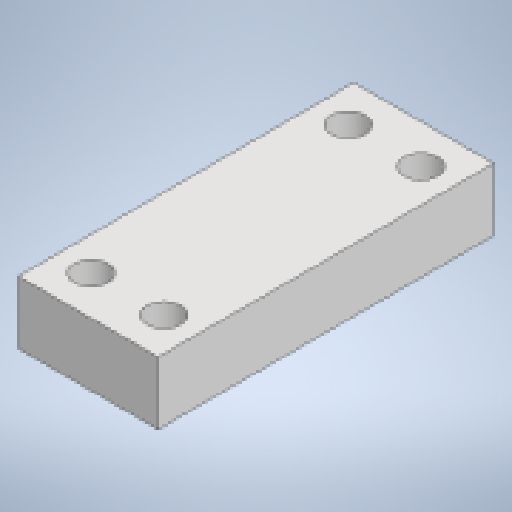
# Autodesk Inventor part: BK10_3030_Mount
Saved by Autodesk Inventor 2023 (Build 270158000, 158)
## iProperties
Created: 2022-04-29
Part Number: BK10_3030_Mount
Material: Generic
Document SubType Name: Modeling
Designer: plebbb
Density: 1 g/cm^3
Appearance: Default
Author: plebbb
Autodesk Inventor part; units mm, degrees
ref_plane "YZ Plane" through (0, 0, 0) normal (1, 0, 0) x (0, 1, 0)
ref_plane "XZ Plane" through (0, 0, 0) normal (0, 1, 0) x (-1, 0, 0)
ref_plane "XY Plane" through (0, 0, 0) normal (0, 0, 1) x (1, 0, 0)
sketch "Sketch1" plane through (0, 0, 0) normal (1, 0, 0) x (0, 1, 0)
  line L0 (0, 0) -> (0, 60)
  line L1 (0, 60) -> (11.2, 60)
  line L2 (11.2, 60) -> (11.2, 0)
  line L3 (11.2, 0) -> (0, 0)
  dimension "d2" = 60
  dimension "d4" = 11.2
  constraints: 8 end point, 2 perpendicular, 1 coincident, 1 vertical
  measures "d2" distance of L1.end L2.end
  measures "d4" distance between parallel lines of L2 L0
extrude "Extrusion1" add sketch "Sketch1" along normal blind 25
sketch "Sketch2" plane through (0, 11.2, 60) normal (0, 1, 0) x (1, 0, 0)
  circle A0 centre (6, 53) radius 3
  point P0 (0, 60)
  dimension "d7" = 6
  dimension "d8" = 6
  dimension "d9" = 7
  constraints: 1 centre point
  measures "d7" diameter of A0
  measures "d8" horizontal distance of point (0, 60) A0.centre
  measures "d9" vertical distance of point (0, 60) A0.centre
extrude "Extrusion2" cut sketch "Sketch2" against normal blind 20
pattern_linear "Rectangular Pattern1" count 2 spacing 46 along (0, 0, 1) count 2 spacing 13 along (1, 0, 0) of "Extrusion2"
body "Solid1"
